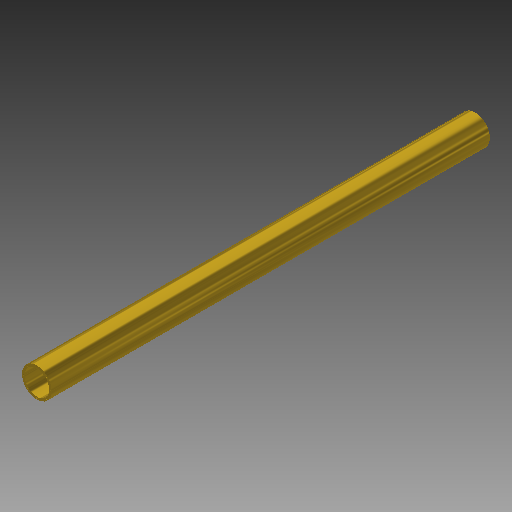
# Autodesk Inventor part: Electrode 3
Saved by Autodesk Inventor 2017 (Build 210142000, 142)
## iProperties
Created: 2009-05-06
Part Number: Electrode 3
Document SubType Name: Modeling
Designer: Serena
Material: Generic
Density: 1 g/cm^3
Appearance: Glossy - Gold
Author: Serena
Autodesk Inventor part; units mm, degrees
ref_plane "YZ Plane" through (0, 0, 0) normal (1, 0, 0) x (0, 1, 0)
ref_plane "XZ Plane" through (0, 0, 0) normal (0, 1, 0) x (-1, 0, 0)
ref_plane "XY Plane" through (0, 0, 0) normal (0, 0, 1) x (1, 0, 0)
sketch "Sketch1" plane through (0, 0, 0) normal (0, 0, 1) x (1, 0, 0)
  circle A0 centre (0, 0) radius 15.25
  circle A1 centre (0, 0) radius 18.25
  dimension "d0" = 30.5
  dimension "d1" = 36.5
  constraints: 2 centre point, 1 coincident
  measures "d0" diameter of A0
  measures "d1" diameter of A1
extrude "Extrusion1" add sketch "Sketch1" along normal blind 539.8
sketch "Sketch2" plane through (0, 0, 0) normal (0, 1, 0) x (-1, 0, 0)
  line L0 (18.25, 0) -> (18.25, 539.8) projected
  line L1 (15.25, 0) -> (15.25, 539.8) projected
  line L2 (-18.25, 539.8) -> (18.25, 539.8) projected
  line L3 (-18.25, 0) -> (18.25, 0) projected
  line L4 (16.75, 539.8) -> (16.75, 484.0456)
  line L5 (16.75, 527.9588) -> (15.25, 527.9588)
  line L6 (16.75, 525.4794) -> (18.25, 525.4794)
  line L7 (16.75, 539.8) -> (16.75, 545.2687)
  circle A0 centre (16.75, 540.3) radius 1
  line L8 (16.75, 539.8) -> (16.75, 539.3)
  line L9 (16.75, 539.8) -> (15.884, 539.8)
  arc A1 (15.884, 539.8) -> (16.75, 539.3) centre (16.75, 540.3) ccw
  dimension "d4" = 2
  dimension "d5" = 0.5
  constraints: 12 end point, 8 point on line, 4 point on circle, 3 perpendicular, 2 centre point, 2 parallel, 1 concentric
  measures "d4" diameter of A0
  measures "d5" distance of L4.start L8.end
revolve "Revolution1" cut sketch "Sketch2" angle 360 about axis through (-16.75, 0, 539.8) along (0, 0, -1) picked at (16.2136, 539.7436) contours L4 A0 L2
pattern_circular "Circular Pattern2" count 8 over 360 about axis through (0, 0, 0) along (0, 0, 1) of "Revolution1"
sketch "Sketch3" plane through (0, 0, 0) normal (0, 1, 0) x (-1, 0, 0)
  line L0 (18.25, 0) -> (18.25, 539.8) projected
  line L1 (15.25, 0) -> (15.25, 539.8) projected
  line L2 (-18.25, 0) -> (18.25, 0) projected
  line L3 (16.75, 0) -> (16.75, 57.9102)
  line L4 (16.75, 9.1086) -> (15.25, 9.1086)
  line L5 (16.75, 7.2128) -> (18.25, 7.2128)
  line L6 (16.75, 0) -> (16.75, -10.4)
  circle A0 centre (16.75, -0.5) radius 1
  line L7 (16.75, 0.5) -> (16.75, 0)
  line L8 (16.75, 0) -> (17.616, 0)
  arc A1 (17.616, 0) -> (16.75, 0.5) centre (16.75, -0.5) ccw
  dimension "d13" = 2
  dimension "d14" = 0.5
  constraints: 12 end point, 8 point on line, 4 point on circle, 3 perpendicular, 2 centre point, 2 parallel, 1 collinear, 1 concentric
  measures "d13" diameter of A0
  measures "d14" distance of L7.start L3.start
revolve "Revolution2" cut sketch "Sketch3" angle 360 about axis through (-16.75, 0, 0) along (0, 0, 1) picked at (17.2864, 0.0564) contours L2 L3 A0
pattern_circular "Circular Pattern3" count 8 over 360 about axis through (0, 0, 0) along (0, 0, 1) of "Revolution2"
body "Solid1"
